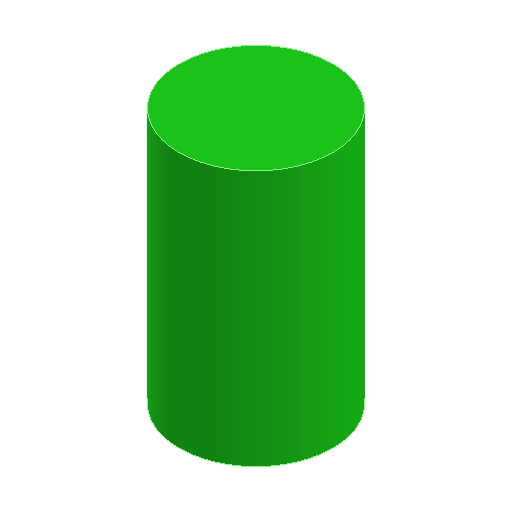
# Autodesk Inventor part: Cylinder
Saved by Autodesk Inventor 2026.1 (Build 301233020, 233B)
## iProperties
Created: 2026-01-20
Part Number: Cylinder
Material: Generic
Document SubType Name: Modeling
Designer: holy
Density: 1 g/cm^3
Appearance: Default
Author: holy
Autodesk Inventor part; units mm, degrees
ref_plane "YZ Plane" through (0, 0, 0) normal (1, 0, 0) x (0, 1, 0)
ref_plane "XZ Plane" through (0, 0, 0) normal (0, 1, 0) x (-1, 0, 0)
ref_plane "XY Plane" through (0, 0, 0) normal (0, 0, 1) x (1, 0, 0)
sketch "Sketch1" plane through (0, 0, 0) normal (0, 0, 1) x (1, 0, 0)
  line L0 (-15.24, 0) -> (91.44, 0) construction
  line L1 (0, -50.8) -> (0, 304.8) construction
  line L2 (76.2, 0) -> (0, 0)
  line L3 (0, 0) -> (0, 254)
  line L4 (0, 254) -> (76.2, 254)
  line L5 (76.2, 254) -> (76.2, 0)
  point P0 (0, 0)
  dimension "d0" = 76.2
  dimension "d1" = 254
  constraints: 8 end point, 2 collinear, 2 parallel, 1 horizontal, 1 perpendicular
  measures "d0" distance of L3.end L4.end
  measures "d1" distance of L4.end L2.start
revolve "Revolution1" add sketch "Sketch1" angle 360 about axis through (0, 0, 0) along (0, 1, 0)
equation "\"d0\" = 0.5 * BaseDia"
equation "\"d1\" = Height"
equation "\"BaseDia\" = 152.4"
equation "\"Height\" = 254"
body "Solid1"
